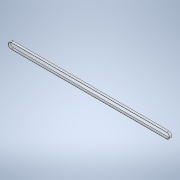
# Autodesk Inventor part: belt
Saved by Autodesk Inventor 2020 (Build 240168000, 168)
## iProperties
Created: 2021-02-26
Part Number: belt
Material: Generic
Document SubType Name: Modeling
Designer: AOB
Mass: 3.24691 g
Surface Area: 113.899 cm^2
Volume: 3.24691 cm^3
Density: 1 g/cm^3
Appearance: Default
Author: AOB
Autodesk Inventor part; units mm, degrees
ref_plane "YZ Plane" through (0, 0, 0) normal (1, 0, 0) x (0, 1, 0)
ref_plane "XZ Plane" through (0, 0, 0) normal (0, 1, 0) x (-1, 0, 0)
ref_plane "XY Plane" through (0, 0, 0) normal (0, 0, 1) x (1, 0, 0)
sketch "Sketch1" plane through (0, 0, 0) normal (0, 0, 1) x (1, 0, 0)
  arc A0 (0, 7.1111) -> (0, -7.1111) centre (0, 0) ccw
  arc A1 (406.155, -7.1111) -> (406.155, 7.1111) centre (406.155, 0) ccw
  line L0 (0, 7.1111) -> (406.155, 7.1111)
  line L1 (406.155, -7.1111) -> (0, -7.1111)
  line L2 (0, 7.1111) -> (0, 7.7411) construction
  arc A2 (0, 7.7411) -> (0, -7.7411) centre (0, 0) ccw
  line L3 (0, -7.7411) -> (406.155, -7.7411)
  arc A3 (406.155, -7.7411) -> (406.155, 7.7411) centre (406.155, 0) ccw
  line L4 (0, 7.7411) -> (406.155, 7.7411)
  point P0 (0.1439, -0.3925)
  point P1 (2.475, -0.3925)
  point P2 (2.4728, -0.3925)
  point P3 (0, -0.3925)
  dimension "d8" = 14.2222
  dimension "d9" = 14.2222
  dimension "d10" = 406.155
  dimension "d11" = 0.63
  constraints: 10 end point, 8 point on circle, 5 tangent, 4 centre point, 1 coincident, 1 concentric, 1 horizontal, 1 parallel, 1 point on line, 1 vertical
  measures "d8" diameter of A0
  measures "d9" diameter of A1
  measures "d10" distance of A1.centre A0.centre
  measures "d11" distance of L0.start L2.end
extrude "Extrusion2" add sketch "Sketch1" along normal blind 6
body "Solid2"
